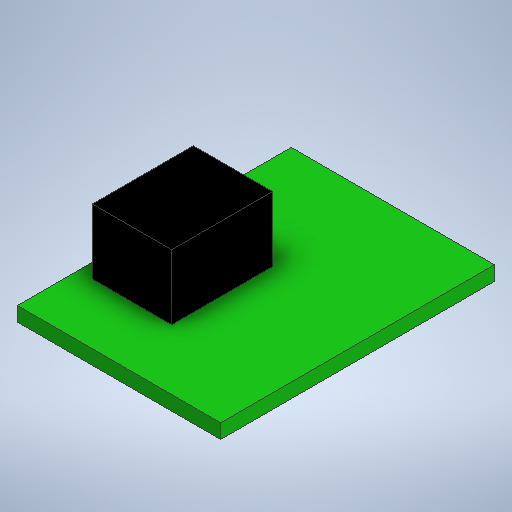
# Autodesk Inventor part: Boost converter
Saved by Autodesk Inventor 2025.2 (Build 292293000, 293)
## iProperties
Created: 2025-04-04
Part Number: Boost converter
Material: Generic
Document SubType Name: Modeling
Designer: joaki
Density: 1 g/cm^3
Appearance: Default
Author: joaki
Autodesk Inventor part; units mm, degrees
ref_plane "YZ Plane" through (0, 0, 0) normal (1, 0, 0) x (0, 1, 0)
ref_plane "XZ Plane" through (0, 0, 0) normal (0, 1, 0) x (-1, 0, 0)
ref_plane "XY Plane" through (0, 0, 0) normal (0, 0, 1) x (1, 0, 0)
sketch "Sketch1" plane through (0, 0, 0) normal (0, 1, 0) x (-1, 0, 0)
  line L0 (5.246, 9.5763) -> (-8.854, 9.5763)
  line L1 (-8.854, 9.5763) -> (-8.854, -9.4237)
  line L2 (-8.854, -9.4237) -> (5.246, -9.4237)
  line L3 (5.246, -9.4237) -> (5.246, 9.5763)
  point P0 (0, 0)
  dimension "d0" = 14.1
  dimension "d1" = 19
  constraints: 8 end point, 2 parallel, 1 horizontal, 1 perpendicular
  measures "d0" distance of L1.end L2.end
  measures "d1" distance of L2.end L0.start
extrude "Extrusion1" add sketch "Sketch1" along normal blind 1
sketch "Sketch2" plane through (0, 1, 0) normal (0, 1, 0) x (1, 0, 0)
  line L0 (-4.246, -5.3763) -> (1.254, -5.3763)
  line L1 (1.254, -5.3763) -> (1.254, 1.6237)
  line L2 (1.254, 1.6237) -> (-4.246, 1.6237)
  line L3 (-4.246, 1.6237) -> (-4.246, -5.3763)
  line L4 (-5.246, 9.4237) -> (-5.246, -9.5763) projected
  line L5 (-5.246, -9.5763) -> (8.854, -9.5763) projected
  point P0 (0, 0)
  point P1 (-1.496, -5.3763)
  dimension "d4" = 5.5
  dimension "d5" = 7
  dimension "d6" = 1
  dimension "d7" = 4.2
  constraints: 8 end point, 2 parallel, 1 horizontal, 1 midpoint, 1 perpendicular
  measures "d4" distance of L1.end L2.end
  measures "d5" distance of L2.end L0.start
  measures "d6" distance between parallel lines of L4 L3
  measures "d7" distance from line of L5 point (-1.496, -5.376)
extrude "Extrusion2" add sketch "Sketch2" along normal blind 4.5
body "Solid1"
